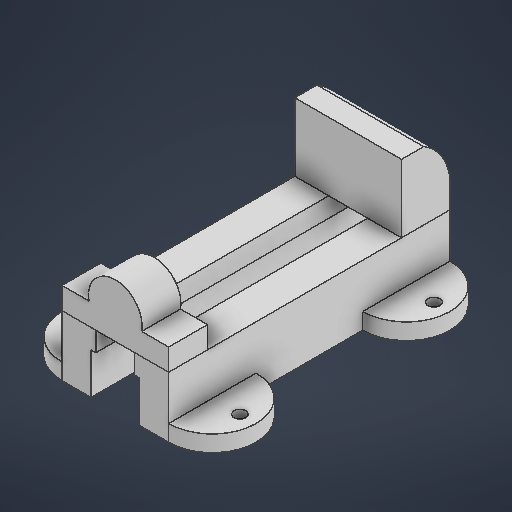
# Autodesk Inventor part: yeni_mengene_ho
Saved by Autodesk Inventor 2025.4 (Build 294407000, 407)
## iProperties
Created: 2026-06-19
Part Number: yeni_mengene_ho
Material: Generic
Document SubType Name: Modeling
Designer: yigithan
Density: 1 g/cm^3
Appearance: Default
Author: yigithan
Autodesk Inventor part; units mm, degrees
ref_plane "YZ Plane" through (0, 0, 0) normal (1, 0, 0) x (0, 1, 0)
sketch "Sketch1" plane through (0, 0, 0) normal (0, 0, 1) x (1, 0, 0)
  line L0 (0, 0) -> (69.85, 0)
  line L1 (69.85, 0) -> (69.85, 39.67)
  line L2 (69.85, 39.67) -> (0, 39.67)
  line L3 (0, 39.67) -> (0, 0)
  dimension "d0" = 69.85
  dimension "d1" = 39.67
  constraints: 8 end point, 2 parallel, 1 horizontal, 1 perpendicular
  measures "d0" distance of L2.end L1.end
  measures "d1" distance of L1.end L0.end
extrude "Extrusion1" add sketch "Sketch1" against normal blind 184.15
sketch "Sketch2" plane through (69.85, 0, 0) normal (1, 0, 0) x (0, 0, -1)
  line L0 (184.15, 39.67) -> (184.15, 0) projected
  line L1 (184.15, 39.67) -> (152.41, 39.67)
  line L2 (0, 39.67) -> (184.15, 39.67) projected
  line L3 (152.41, 39.67) -> (152.41, 84.12)
  line L4 (152.41, 39.67) -> (196.86, 39.67) construction
  line L5 (152.41, 84.12) -> (166.86, 84.12)
  arc A0 (184.15, 53.97) -> (166.8575, 84.12) centre (149.22, 53.97) ccw
  line L6 (184.15, 39.67) -> (184.15, 53.97)
  point P0 (0, 0)
  dimension "d4" = 31.74
  dimension "d5" = 44.45
  dimension "d6" = 90
  dimension "d7" = 14.45
  dimension "d8" = 90
  dimension "d9" = 69.86
  dimension "d10" = 30.15
  constraints: 10 end point, 3 perpendicular, 2 point on circle, 2 point on line, 1 centre point, 1 horizontal, 1 tangent, 1 vertical
  measures "d4" distance of L0.start L1.end
  measures "d5" distance of L1.end L3.end
  measures "d6" angle of L4 L3
  measures "d7" distance of L3.end L5.end
  measures "d8" angle of L3 L5
  measures "d9" diameter of A0
  measures "d10" distance from line of L5 A0.centre
extrude "Extrusion2" add sketch "Sketch2" against normal blind 69.85 separate body
sketch "Sketch3" plane through (0, 0, 0) normal (0, 0, 1) x (1, 0, 0)
  line L0 (69.85, 84.12) -> (0, 84.12) projected
  line L1 (0, 39.67) -> (69.85, 39.67) projected
  line L2 (0, 84.12) -> (0, 53.97) projected
  line L3 (0, 53.97) -> (0, 39.67)
  line L4 (69.85, 39.67) -> (69.85, 0) projected
  line L5 (69.85, 53.97) -> (69.85, 39.67)
  line L6 (0, 53.97) -> (0, 39.67) projected
  line L7 (0, 39.67) -> (0, 53.97)
  line L8 (69.85, 53.97) -> (0, 53.97) projected
  line L9 (69.85, 53.97) -> (69.85, 39.67)
  arc A0 (52.1642, 53.97) -> (17.6858, 53.97) centre (34.925, 57.15) ccw
  arc A1 (33.6019, 39.67) -> (36.2481, 39.67) centre (34.925, 57.15) ccw
  line L10 (0, 53.97) -> (17.6858, 53.97)
  line L11 (52.1642, 53.97) -> (69.85, 53.97)
  point P0 (0, 0)
  point P1 (17.6858, 53.97)
  dimension "d14" = 17.48
  constraints: 12 end point, 4 point on circle, 2 centre point, 2 collinear, 2 perpendicular, 2 point on line
  measures "d14" distance from line of L1 A0.centre
extrude "Extrusion3" add sketch "Sketch3" against normal blind 25.4 separate body contours L3 L8 L5 L1 | A0 L8
sketch "Sketch4" plane through (0, 0, 0) normal (0, 0, 1) x (1, 0, 0)
  line L0 (22.225, 42.93) -> (47.625, 42.93)
  line L1 (0, 0) -> (69.85, 0) projected
  line L2 (22.225, 42.93) -> (22.225, 26.92)
  line L3 (22.225, 26.92) -> (19.045, 26.92)
  line L4 (19.045, 26.92) -> (19.045, 0)
  line L5 (34.925, 0) -> (34.925, 13.46)
  line L6 (47.625, 42.93) -> (47.625, 26.92)
  line L7 (47.625, 26.92) -> (50.805, 26.92)
  line L8 (50.805, 26.92) -> (50.805, 0)
  line L9 (19.045, 0) -> (19.045, -11.3598)
  line L10 (19.045, -11.3598) -> (50.805, -11.3598)
  line L11 (50.805, -11.3598) -> (50.805, 0)
  point P0 (34.925, 42.93)
  dimension "d17" = 25.4
  dimension "d18" = 16.01
  dimension "d19" = 3.18
  dimension "d20" = 26.92
  constraints: 22 end point, 4 perpendicular, 3 midpoint, 3 symmetric about line, 3 vertical, 1 horizontal, 1 vertical alignment
  measures "d17" distance of L0.start L0.end
  measures "d18" distance of L0.start L2.end
  measures "d19" distance of L2.end L3.end
  measures "d20" distance of L3.end L4.end
extrude "Extrusion4" cut sketch "Sketch4" against normal blind 319.9 contours L0 L6 L7 L8 L1 L4 L3 L2 bodies 1
sketch "Sketch5" plane through (69.85, 0, -184.15) normal (0, -1, 0) x (1, 0, 0)
  line L0 (0, 184.15) -> (-17.6858, 184.15) projected
  line L1 (0, 184.15) -> (0, 155.57)
  line L2 (0, 184.15) -> (0, 158.75) projected
  arc A0 (0, 126.99) -> (0, 184.15) centre (0, 155.57) ccw
  circle A1 centre (18, 155.57) radius 3.96
  line L3 (0, 184.15) -> (0, 126.99)
  point P0 (-69.85, 184.15)
  constraints: 4 end point, 2 centre point, 2 point on circle, 1 coincident, 1 collinear, 1 point on line
extrude "Extrusion5" add sketch "Sketch5" against normal blind 10.6 bodies 1
ref_plane "Work Plane1" through (34.925, 0, -184.15) normal (1, 0, 0) x (0, 0, -1)
ref_plane "Work Plane2" through (0, 0, -92.075) normal (0, 0, -1) x (-1, 0, 0)
mirror "Mirror2" about plane through (0, 0, -92.075) normal (0, 0, -1) of "Extrusion5" bodies 1
mirror "Mirror3" about plane through (34.925, 0, -184.15) normal (1, 0, 0) of "Extrusion5", "Mirror2" bodies 1
body "Solid1"
body "Solid2"
body "Solid3"
